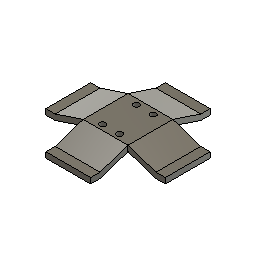
sarvo_dai v1 (Autodesk Fusion 360 design; units mm, degrees)
Autodesk Fusion 360 part; units mm, degrees
sketch "スケッチ1" plane through (0, 0, 0) normal (0, 1, 0) x (1, 0, 0)
  line L0 (12, 12) -> (-12, 12)
  line L1 (-12, 12) -> (-12, -12)
  line L2 (-12, -12) -> (12, -12)
  line L3 (12, -12) -> (12, 12)
  line L4 (12, 12) -> (-12, -12) construction
  line L5 (-12, 12) -> (12, -12) construction
  line L6 (4.5, 9) -> (-4.5, 9)
  line L7 (-4.5, 9) -> (-4.5, -9)
  line L8 (-4.5, -9) -> (4.5, -9)
  line L9 (4.5, -9) -> (4.5, 9)
  line L10 (4.5, 9) -> (-4.5, -9) construction
  line L11 (-4.5, 9) -> (4.5, -9) construction
  circle A0 centre (-4.5, 9) radius 1.6
  circle A1 centre (4.5, 9) radius 1.6
  circle A2 centre (-4.5, -9) radius 1.6
  circle A3 centre (4.5, -9) radius 1.6
  dimension "d1" = 24
  dimension "d2" = 24
  dimension "d3" = 9
  dimension "d4" = 18
  dimension "d5" = 3.2
  dimension "d6" = 3.2
  dimension "d7" = 3.2
  dimension "d8" = 3.2
  constraint perpendicular L0 L1
  constraint parallel L0 L2
  constraint parallel L1 L3
  constraint horizontal L0
  constraint coincident L4 origin
  constraint coincident L5 origin
  constraint perpendicular L6 L7
  constraint parallel L6 L8
  constraint parallel L7 L9
  constraint horizontal L6
  constraint coincident L10 origin
  constraint coincident L11 origin
  constraint coincident L6.end L7.start
  constraint coincident L6.start L9.end
  constraint coincident L7.end L8.start
  constraint coincident L8.end L9.start
  measures "d1" distance of L0.end L1.end
  measures "d2" distance of L1.end L2.end
  measures "d3" distance of L7.end L8.end
  measures "d4" distance of L6.end L7.end
  measures "d5" diameter of A0
  measures "d6" diameter of A1
  measures "d7" diameter of A2
  measures "d8" diameter of A3
extrude "押し出し1" add sketch "スケッチ1" along normal blind 3 contours L0 L1 L2 L3 | L6 L7 L8 L9 A0 A1 A2 A3
sketch "スケッチ2" plane through (0, 0, 0) normal (0, 0, 1) x (1, 0, 0)
  line L0 (12, 0) -> (12, -5)
  line L1 (12, -5) -> (27, -5)
  line L2 (27, -5) -> (12, 0)
  line L3 (27, -5) -> (27, -2)
  line L4 (27, -2) -> (12, 3)
  line L5 (12, 0) -> (12, 3)
  line L6 (27, -2) -> (32, -2)
  line L7 (32, -2) -> (32, -5)
  line L8 (32, -5) -> (27, -5)
  line L9 (27, -5) -> (27, -2)
  dimension "d11" = 5
  dimension "d12" = 15
  dimension "d13" = 3
  dimension "d14" = 5
  dimension "d15" = 3
  constraint vertical L0
  constraint perpendicular L0 L1
  constraint perpendicular L1 L3
  constraint parallel L0 L5
  constraint horizontal L6
  constraint vertical L7
  constraint horizontal L8
  constraint vertical L9
  measures "d11" distance of L0.start L0.end
  measures "d12" distance of L0.end L1.end
  measures "d13" distance of L1.end L3.end
  measures "d14" distance of L3.end L6.end
  measures "d15" distance of L3.end L1.end
extrude "押し出し2" add sketch "スケッチ2" along normal mid plane 24 contours L2 L3 L4 L5 L9 | L3 L6 L7 L8 L9
sketch "スケッチ3" plane through (0, 0, 0) normal (0, 0, 1) x (1, 0, 0)
  line L0 (-12, 0) -> (-12, -5)
  line L1 (-12, -5) -> (-27, -5)
  line L2 (-12, 0) -> (-27, -5)
  line L3 (-27, -5) -> (-27, -2)
  line L4 (-27, -2) -> (-12, 3)
  line L5 (-12, 3) -> (-12, 0)
  line L6 (-27, -2) -> (-32, -2)
  line L7 (-32, -2) -> (-32, -5)
  line L8 (-32, -5) -> (-27, -5)
  line L9 (-27, -5) -> (-27, -2)
  dimension "d18" = 5
  dimension "d19" = 15
  dimension "d20" = 3
  dimension "d21" = 5
  dimension "d22" = 3
  constraint vertical L0
  constraint perpendicular L0 L1
  constraint perpendicular L1 L3
  constraint horizontal L6
  constraint vertical L7
  constraint horizontal L8
  constraint vertical L9
  measures "d18" distance of L0.start L0.end
  measures "d19" distance of L0.end L1.end
  measures "d20" distance of L1.end L3.end
  measures "d21" distance of L3.end L6.end
  measures "d22" distance of L3.end L1.end
extrude "押し出し3" add sketch "スケッチ3" along normal mid plane 24 contours L2 L3 L4 L5 L9 | L3 L6 L7 L8 L9
sketch "スケッチ4" plane through (0, 0, 0) normal (1, 0, 0) x (0, 0, -1)
  line L0 (12, 0) -> (12, -5)
  line L1 (12, -5) -> (27, -5)
  line L2 (27, -5) -> (12, 0)
  line L3 (27, -5) -> (27, -2)
  line L4 (27, -2) -> (12, 3)
  line L5 (12, 3) -> (12, 0)
  line L6 (27, -2) -> (32, -2)
  line L7 (32, -2) -> (32, -5)
  line L8 (32, -5) -> (27, -5)
  line L9 (27, -5) -> (27, -2)
  line L10 (0, 5) -> (0, 4)
  line L11 (0, 4) -> (0, -9)
  line L12 (-27, -2) -> (-12, 3)
  line L13 (-12, 3) -> (-12, 0)
  line L14 (-27, -5) -> (-12, 0)
  line L15 (-27, -2) -> (-32, -2)
  line L16 (-27, -5) -> (-27, -2)
  line L17 (-32, -2) -> (-32, -5)
  line L18 (-32, -5) -> (-27, -5)
  dimension "d25" = 15
  dimension "d26" = 3
  dimension "d27" = 3
  dimension "d28" = 5
  constraint vertical L0
  constraint perpendicular L0 L1
  constraint vertical L3
  constraint parallel L0 L5
  constraint horizontal L6
  constraint vertical L7
  constraint horizontal L8
  constraint vertical L9
  constraint vertical L10
  constraint parallel L10 L11
  constraint symmetric L0.start L11 L13.end
  constraint symmetric L1.end L11 L14.start
  constraint symmetric L3.end L11 L12.start
  constraint symmetric L4.end L11 L12.end
  constraint symmetric L6.end L11 L15.end
  constraint symmetric L7.end L11 L17.end
  measures "d25" distance of L0.end L1.end
  measures "d26" distance of L1.end L3.end
  measures "d27" distance of L3.end L1.end
  measures "d28" distance of L3.end L6.end
extrude "押し出し4" add sketch "スケッチ4" along normal mid plane 24 contours L2 L3 L4 L5 L9 | L3 L6 L7 L8 L9 | L15 L16 L17 L18 | L12 L13 L14 L16
